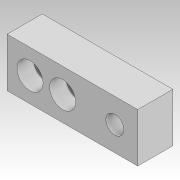
# Autodesk Inventor part: LoadCellMount
Saved by Autodesk Inventor 2020 (Build 240168000, 168)
## iProperties
Created: 2022-01-26
Part Number: LoadCellMount
Material: Generic
Document SubType Name: Modeling
Designer: DDeGo
Density: 1 g/cm^3
Appearance: Default
Author: DDeGo
Autodesk Inventor part; units mm, degrees
ref_plane "YZ Plane" through (0, 0, 0) normal (1, 0, 0) x (0, 1, 0)
ref_plane "XZ Plane" through (0, 0, 0) normal (0, 1, 0) x (-1, 0, 0)
ref_plane "XY Plane" through (0, 0, 0) normal (0, 0, 1) x (1, 0, 0)
sketch "Sketch1" plane through (0, 0, 0) normal (0, 0, 1) x (1, 0, 0)
  line L0 (-20, -7.5) -> (20, -7.5)
  line L1 (20, -7.5) -> (20, 7.5)
  line L2 (20, 7.5) -> (-20, 7.5)
  line L3 (-20, 7.5) -> (-20, -7.5)
  line L4 (-20, -7.5) -> (20, 7.5) construction
  line L5 (20, -7.5) -> (-20, 7.5) construction
  point P0 (0, 0)
  dimension "d0" = 15
  dimension "d1" = 40
  constraints: 12 end point, 2 midpoint, 2 parallel, 1 horizontal, 1 perpendicular
  measures "d0" distance of L2.end L0.start
  measures "d1" distance of L1.end L2.end
extrude "Extrusion1" add sketch "Sketch1" along normal blind 10.75
sketch "Sketch2" plane through (0, 0, 10.75) normal (0, 0, 1) x (1, 0, 0)
  line L0 (-20, 7.5) -> (-20, -7.5) construction
  line L1 (-20, 0) -> (-13, 0) construction
  line L2 (-13, 0) -> (-3, 0) construction
  circle A0 centre (-13, 0) radius 2.25
  circle A1 centre (-3, 0) radius 2.25
  point P0 (0, 0)
  dimension "d4" = 10
  dimension "d5" = 7
  dimension "d6" = 4.5
  constraints: 4 end point, 2 centre point, 2 coincident, 1 equal radius, 1 horizontal, 1 midpoint, 1 point on line
  measures "d4" distance of L1.end L2.end
  measures "d5" distance of L1.start L1.end
  measures "d6" diameter of A0
extrude "Extrusion2" cut sketch "Sketch2" against normal through all
sketch "Sketch3" plane through (0, 0, 10.75) normal (0, 0, 1) x (1, 0, 0)
  circle A0 centre (-13, 0) radius 2.25 projected
  circle A1 centre (-13, 0) radius 4
  circle A2 centre (-3, 0) radius 2.25 projected
  circle A3 centre (-3, 0) radius 4
  point P0 (0, 0)
  dimension "d9" = 8
  constraints: 2 centre point, 2 coincident, 1 equal radius
  measures "d9" diameter of A1
extrude "Extrusion3" cut sketch "Sketch3" against normal blind 5 contours A0 | A1 | A2 | A3
sketch "Sketch4" plane through (0, 0, 0) normal (0, 0, -1) x (-1, 0, 0)
  line L0 (-20, -7.5) -> (-20, 7.5) construction
  line L1 (-20, 0) -> (-13, 0) construction
  circle A0 centre (-13, 0) radius 2.75
  point P0 (0, 0)
  dimension "d12" = 5.5
  dimension "d13" = 7
  constraints: 2 end point, 1 centre point, 1 coincident, 1 horizontal, 1 midpoint
  measures "d12" diameter of A0
  measures "d13" distance of L1.start L1.end
extrude "Extrusion4" cut sketch "Sketch4" against normal through all
sketch "Sketch5" plane through (0, 0, 0) normal (0, 0, -1) x (-1, 0, 0)
  circle A0 centre (-13, 0) radius 2.75 projected
  circle A1 centre (-13, 0) radius 4.75
  point P0 (0, 0)
  dimension "d16" = 9.5
  constraints: 1 centre point, 1 coincident
  measures "d16" diameter of A1
extrude "Extrusion5" cut sketch "Sketch5" against normal blind 6 contours A0 | A1
body "Solid1"
